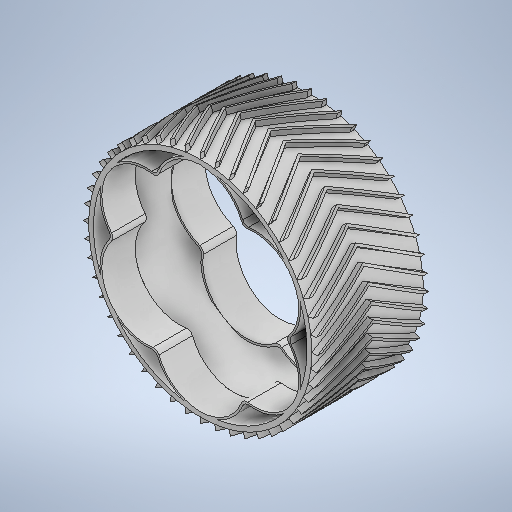
# Autodesk Inventor part: opona_nowa
Saved by Autodesk Inventor 2025.2 (Build 292293000, 293)
## iProperties
Created: 2026-03-13
Part Number: opona_nowa
Material: Generic
Document SubType Name: Modeling
Designer: ksawe
Density: 1 g/cm^3
Appearance: Default
Author: ksawe
Autodesk Inventor part; units mm, degrees
ref_plane "YZ Plane" through (0, 0, 0) normal (1, 0, 0) x (0, 1, 0)
ref_plane "XY Plane" through (0, 0, 0) normal (0, 0, 1) x (1, 0, 0)
sketch "Sketch1" plane through (0, 0, 0) normal (0, 0, 1) x (1, 0, 0)
  circle A0 centre (0, 0) radius 60
  circle A1 centre (0, 0) radius 57.5
  dimension "d0" = 120
  dimension "d1" = 115
  constraints: 2 centre point, 2 coincident
  measures "d0" diameter of A0
  measures "d1" diameter of A1
extrude "Extrusion1" add sketch "Sketch1" along normal mid plane 60
sketch "Sketch2" plane through (0, 0, 30) normal (0, 0, 1) x (1, 0, 0)
  circle A0 centre (0, 0) radius 47.5
  circle A1 centre (0, 0) radius 57.5 projected
  line L0 (0, 0) -> (47.5, 0) construction
  line L1 (0, 0) -> (47.5, 0) construction
  circle A2 centre (0, 0) radius 46 construction
  line L2 (0, 0) -> (23, 39.8372) construction
  line L3 (0, 0) -> (46, 0) construction
  line L4 (0, 0) -> (-23, 39.8372) construction
  line L5 (0, 0) -> (46, 0) construction
  arc A3 (23, 39.8372) -> (-23, 39.8372) centre (0, 33.6936) ccw
  arc A4 (23.9661, 40.0952) -> (-23.9661, 40.0952) centre (0, 33.6936) ccw
  arc A5 (-22.7404, 40.8029) -> (-46.7066, -0.7077) centre (-29.1795, 16.8468) ccw
  arc A6 (-23, 39.8372) -> (-46, 0) centre (-29.1795, 16.8468) ccw
  arc A7 (-46.7066, 0.7077) -> (-22.7404, -40.8029) centre (-29.1795, -16.8468) ccw
  arc A8 (-46, 0) -> (-23, -39.8372) centre (-29.1795, -16.8468) ccw
  arc A9 (-23.9661, -40.0952) -> (23.9661, -40.0952) centre (0, -33.6936) ccw
  arc A10 (-23, -39.8372) -> (23, -39.8372) centre (0, -33.6936) ccw
  arc A11 (22.7404, -40.8029) -> (46.7066, 0.7077) centre (29.1795, -16.8468) ccw
  arc A12 (23, -39.8372) -> (46, 0) centre (29.1795, -16.8468) ccw
  arc A13 (46.7066, -0.7077) -> (22.7404, 40.8029) centre (29.1795, 16.8468) ccw
  arc A14 (46, 0) -> (23, 39.8372) centre (29.1795, 16.8468) ccw
  point P0 (47.4998, 0.1219)
  point P1 (53.7115, 20.5261)
  point P2 (44.6319, 36.2525)
  point P3 (23.8555, 41.0751)
  point P4 (23.6443, 41.197)
  point P5 (9.0796, 56.7786)
  point P6 (0, 57.5)
  point P7 (23, 39.8372)
  point P8 (25.1322, 40.3066)
  point P9 (47.4726, 1.6118)
  point P10 (46, 0)
  point P11 (49.7965, -28.75)
  point P12 (53.7115, -20.5261)
  point P13 (47.4998, -0.1219)
  point P14 (0, -57.5)
  point P15 (9.0796, -56.7786)
  point P16 (23.6443, -41.197)
  point P17 (23.8555, -41.0751)
  point P18 (44.6319, -36.2525)
  point P19 (-49.7965, -28.75)
  point P20 (-44.6319, -36.2525)
  point P21 (-23.8555, -41.0751)
  point P22 (-23.6443, -41.197)
  point P23 (-9.0796, -56.7786)
  point P24 (-49.7965, 28.75)
  point P25 (-53.7115, 20.5261)
  point P26 (-47.4998, 0.1219)
  point P27 (-47.4998, -0.1219)
  point P28 (-53.7115, -20.5261)
  point P29 (-9.0796, 56.7786)
  point P30 (-23.6443, 41.197)
  point P31 (-23.8555, 41.0751)
  point P32 (-44.6319, 36.2525)
  point P33 (49.7965, 28.75)
  point P34 (23.6939, 41.039)
  point P35 (23.6939, -41.039)
  point P36 (47.3878, 0)
  point P37 (-23.6939, -41.039)
  point P38 (-47.3878, 0)
  point P39 (-23.6939, 41.039)
  dimension "d4" = 95
  dimension "d122" = 92
  dimension "d123" = 60
  dimension "d124" = 120
  dimension "d129" = 1
  dimension "d132" = 360
  constraints: 26 point on circle, 14 centre point, 12 end point, 4 coincident, 4 horizontal, 2 equal length, 43 other
  measures "d4" diameter of A0
  measures "d122" diameter of A2
  measures "d123" angle of L3 L2
  measures "d124" angle of L5 L4
  measures "d129" radial gap between concentric circles of A3 A4
extrude "Extrusion3" add sketch "Sketch2" against normal blind 18 contours A13 A11 A0 A12 A14 | A0 A14 A1 A13 | A11 A1 A12 A0 | A14 A3 A0 A4 A13 | A0 A13 A1 A14 | A12 A1 A11 A0 | A0 A11 A9 A10 A12 | A4 A0 A3 A1 | A1 A10 A0 A9 | A3 A0 A4 A1 | A1 A9 A0 A10 | A3 A6 A0 A5 A4 | A5 A0 A6 A1 | A0 A9 A7 A8 A10 | A1 A8 A0 A7 | A6 A0 A5 A1 | A1 A7 A0 A8 | A6 A8 A0 A7 A5
fillet "Fillet2" radius 3 1 edges at (-23, 39.8372, 21)
fillet "Fillet3" radius 3 5 edges at (23, 39.8372, 21) (46, 0, 21) (23, -39.8372, 21) (-23, -39.8372, 21) (-46, 0, 21)
fillet "Fillet4" radius 3 6 edges at (-23.6939, 41.039, 21) (23.6939, 41.039, 21) (47.3878, 0, 21) (23.6939, -41.039, 21) (-23.6939, -41.039, 21) (-47.3878, 0, 21)
sketch "Sketch6" plane through (0, 0, -30) normal (0, 0, -1) x (-1, 0, 0)
  circle A0 centre (0, 0) radius 47.5
  line L0 (0, 0) -> (47.5, 0) construction
  line L1 (0, 0) -> (47.5, 0) construction
  circle A1 centre (0, 0) radius 46 construction
  line L2 (0, 0) -> (39.8372, 23) construction
  line L3 (0, 0) -> (46, 0) construction
  line L4 (0, 0) -> (0, 46) construction
  line L5 (0, 0) -> (46, 0) construction
  arc A2 (39.8372, 23) -> (0, 46) centre (16.8468, 29.1795) ccw
  arc A3 (40.8029, 22.7404) -> (-0.7077, 46.7066) centre (16.8468, 29.1795) ccw
  arc A4 (0.7077, 46.7066) -> (-40.8029, 22.7404) centre (-16.8468, 29.1795) ccw
  arc A5 (0, 46) -> (-39.8372, 23) centre (-16.8468, 29.1795) ccw
  arc A6 (-40.0952, 23.9661) -> (-40.0952, -23.9661) centre (-33.6936, 0) ccw
  arc A7 (-39.8372, 23) -> (-39.8372, -23) centre (-33.6936, 0) ccw
  arc A8 (-40.8029, -22.7404) -> (0.7077, -46.7066) centre (-16.8468, -29.1795) ccw
  arc A9 (-39.8372, -23) -> (0, -46) centre (-16.8468, -29.1795) ccw
  arc A10 (-0.7077, -46.7066) -> (40.8029, -22.7404) centre (16.8468, -29.1795) ccw
  arc A11 (0, -46) -> (39.8372, -23) centre (16.8468, -29.1795) ccw
  arc A12 (40.0952, -23.9661) -> (40.0952, 23.9661) centre (33.6936, 0) ccw
  arc A13 (39.8372, -23) -> (39.8372, 23) centre (33.6936, 0) ccw
  point P0 (0, 47.3878)
  point P1 (-41.039, 23.6939)
  point P2 (-41.039, -23.6939)
  point P3 (0, -47.3878)
  point P4 (41.039, -23.6939)
  point P5 (41.039, 23.6939)
  point P6 (0, -46)
  point P7 (-39.8372, -23)
  point P8 (-39.8372, 23)
  point P9 (0, 46)
  dimension "d139" = 95
  dimension "d140" = 92
  dimension "d141" = 30
  dimension "d142" = 90
  dimension "d145" = 1
  dimension "d148" = 360
  constraints: 26 point on circle, 14 centre point, 12 end point, 4 horizontal, 3 coincident, 2 equal length, 43 other
  measures "d139" diameter of A0
  measures "d140" diameter of A1
  measures "d141" angle of L3 L2
  measures "d142" angle of L5 L4
  measures "d145" radial gap between concentric circles of A2 A3
extrude "Extrusion6" add sketch "Sketch6" against normal blind 18 contours A13 A2 A0 A3 A12 | A0 A12 A13 | A0 A12 A10 A11 A13 | A0 A2 A3 | A10 A0 A11 | A0 A2 A5 A4 A3 | A10 A8 A0 A9 A11 | A0 A5 A4 | A8 A0 A9 | A0 A5 A7 A6 A4 | A8 A6 A0 A7 A9 | A0 A7 A6
fillet "Fillet5" radius 3 12 edges at (39.8372, -23, -21) (39.8372, 23, -21) (0, 46, -21) (-39.8372, 23, -21) (-39.8372, -23, -21) (0, -46, -21) (0, -47.3878, -21) (41.039, -23.6939, -21) (41.039, 23.6939, -21) (0, 47.3878, -21) (-41.039, 23.6939, -21) (-41.039, -23.6939, -21)
ref_plane "Płaszczyzna konstrukcyjna1" through (0, 60, 0) normal (0, 1, 0) x (-1, 0, 0)
sketch "Szkic7" plane through (0, 60, 0) normal (0, 1, 0) x (-1, 0, 0)
  line L0 (20.5261, -30) -> (-20.5261, -30) projected
  line L1 (0, -30) -> (17.3205, 0)
  line L2 (17.3205, 0) -> (0, 30)
  line L3 (-22.2157, 30) -> (22.2157, 30) projected
  line L4 (0, -30) -> (0, -27.5)
  line L5 (0, -27.5) -> (15.8771, 0)
  line L6 (15.8771, 0) -> (0, 27.5)
  line L7 (0, 27.5) -> (0, 30)
  line L8 (17.3205, 0) -> (17.3205, 22.906) construction
  point P0 (0, 0)
  dimension "d153" = -30
  dimension "d155" = 2.5
  constraints: 14 end point, 3 equal length, 2 midpoint, 2 vertical, 1 collinear, 1 parallel, 1 point on line
  measures "d153" angle of L2 L8
  measures "d155" distance of L6.end L2.end
emboss "Wypukłość1" sketch "Szkic7" operation add depth 3 direction (0, -1, 0) wrap yes faces at (59.5708, -7.1637, -10)
pattern_circular "Szyk kołowy3" count 48 over 360 about axis through (0, 0, 0) along (0, 0, 1) of "Wypukłość1"
body "Solid1"
